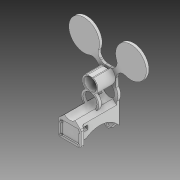
# Autodesk Inventor part: VisionMount
Saved by Autodesk Inventor 2020 (Build 240168000, 168)
## iProperties
Created: 2020-09-30
Part Number: VisionMount
Material: Generic
Document SubType Name: Modeling
Designer: DDeGo
Density: 1 g/cm^3
Appearance: Default
Author: DDeGo
Autodesk Inventor part; units mm, degrees
ref_plane "YZ Plane" through (0, 0, 0) normal (1, 0, 0) x (0, 1, 0)
ref_plane "XZ Plane" through (0, 0, 0) normal (0, 1, 0) x (-1, 0, 0)
ref_plane "XY Plane" through (0, 0, 0) normal (0, 0, 1) x (1, 0, 0)
sketch "Sketch1" plane through (0, 0, 0) normal (0, 0, 1) x (1, 0, 0)
  line L0 (-9.525, 7.14375) -> (-9.525, 19.84375)
  arc A0 (-9.525, 7.14375) -> (-10.31875, -5.939881) centre (0, 0) ccw
  line L1 (-10.31875, -5.939881) -> (-10.31875, -32.816122)
  line L2 (10.31875, -32.816122) -> (10.31875, -5.939881)
  arc A1 (10.31875, -5.939881) -> (9.525, 7.14375) centre (0, 0) ccw
  line L3 (9.525, 19.84375) -> (9.525, 7.14375)
  line L4 (5.55625, 23.8125) -> (9.525, 19.84375)
  line L5 (-9.525, 19.84375) -> (-5.55625, 23.8125)
  line L6 (-5.55625, 23.8125) -> (5.55625, 23.8125)
  line L7 (-10.31875, -32.816122) -> (10.31875, -32.816122)
  arc A2 (-9.525, 7.14375) -> (-10.31875, -5.939881) centre (0, 0) ccw
  arc A3 (10.31875, -5.939881) -> (9.525, 7.14375) centre (0, 0) ccw
  line L8 (0, -32.816122) -> (0, -23.019122) construction
  circle A4 centre (0, -23.019122) radius 2.75 construction
  circle A5 centre (0, 0) radius 8.05
  line L9 (-9.525, 7.14375) -> (10.31875, -5.939881) construction
  line L10 (-10.31875, -5.939881) -> (9.525, 7.14375) construction
  line L11 (9.525, 7.14375) -> (-9.525, 7.14375) construction
  line L12 (-10.31875, -5.939881) -> (10.31875, -5.939881) construction
  line L13 (-9.525, 19.84375) -> (9.525, 19.84375) construction
  line L14 (0, 0.863607) -> (0, 0) construction
  dimension "d0" = 20.6375
  dimension "d2" = 32.81612
  dimension "d3" = 23.8125
  dimension "d4" = 3.96875
  dimension "d5" = 19.05
  dimension "d6" = 9.797
  dimension "d7" = 5.5
  dimension "d8" = 16.1
  dimension "d69" = 11.90625
  dimension "d70" = 45
  dimension "d71" = 45
  dimension "d72" = 26.87624
  constraints: 30 end point, 8 point on circle, 6 centre point, 4 coincident, 4 horizontal, 4 vertical, 2 point on line, 1 concentric, 1 equal length, 1 midpoint, 1 parallel
  measures "d0" distance between parallel lines of L2 L1
  measures "d2" distance from line of L14.end L7
  measures "d3" distance from line of L6 L14.end
  measures "d4" distance from line of L6 L3.start
  measures "d5" distance between parallel lines of L3 L0
  measures "d6" distance of L8.start L8.end
  measures "d7" diameter of A4
  measures "d8" diameter of A5
  measures "d69" radius of A1
  measures "d70" angle of L13 L5
  measures "d71" angle of L13 L4
  measures "d72" distance between parallel lines of L7 L12
extrude "Extrusion1" add sketch "Sketch1" along normal blind 3
sketch "Sketch2" plane through (0, 0, 3) normal (0, 0, 1) x (1, 0, 0)
  line L0 (5.55625, 23.8125) -> (-5.55625, 23.8125)
  line L1 (0, 23.8125) -> (0, 15.8125) construction
  circle A0 centre (0, 15.8125) radius 7.05
  circle A1 centre (0, 0) radius 8.05
  arc A2 (-4.123106, 23.8125) -> (-3.182788, 7.394076) centre (0, 15.8125) ccw
  arc A3 (3.182788, 7.394076) -> (4.123106, 23.8125) centre (0, 15.8125) ccw
  point P0 (0, 0)
  dimension "d11" = 14.1
  dimension "d13" = 8
  dimension "d14" = 9
  constraints: 6 point on circle, 3 centre point, 2 coincident, 2 end point, 2 point on line, 1 concentric, 1 midpoint, 1 vertical
  measures "d11" diameter of A0
  measures "d13" distance of L1.start L1.end
  measures "d14" radius of A3
extrude "Extrusion2" add sketch "Sketch2" along normal blind 20 contours A3 A1 A2 L0
sketch "Sketch3" plane through (10.31875, -32.816122, 0) normal (1, 0, 0) x (0, 0, -1)
  line L0 (-3, 0) -> (-3, 26.876241)
  line L1 (-3, 5) -> (0, 2)
  line L2 (0, 0) -> (0, 26.876241)
  line L3 (0, 0) -> (-3, 0)
  line L4 (0, 2) -> (0, 0)
  line L5 (0, 0) -> (-3, 0)
  line L6 (-3, 5) -> (-3, 0)
  line L7 (-3, 7.047) -> (-3, 12.547)
  point P0 (0, 32.816122)
  dimension "d17" = 45
  dimension "d18" = 2
  constraints: 8 end point, 2 point on line, 1 collinear, 1 perpendicular, 1 vertical
  measures "d17" angle of L0 L1
  measures "d18" distance from line of L3 L1.end
extrude "Extrusion3" cut sketch "Sketch3" against normal through all
sketch "Sketch4" plane through (-5.55625, 23.8125, 0) normal (0, 1, 0) x (1, 0, 0)
  line L0 (13.60625, -3) -> (-2.49375, -3)
  line L1 (2.433144, -3) -> (8.679356, -3)
  line L2 (8.679356, -3) -> (8.679356, -5.5)
  line L3 (8.679356, -5.5) -> (2.433144, -5.5)
  line L4 (2.433144, -5.5) -> (2.433144, -3)
  line L5 (1.433144, -3) -> (1.433144, -23)
  line L6 (9.679356, -3) -> (9.679356, -23)
  point P0 (5.55625, 0)
  point P1 (8.739038, -3)
  point P2 (2.373462, -3)
  dimension "d21" = 1
  dimension "d22" = 1
  dimension "d23" = 2.5
  constraints: 8 end point, 2 parallel, 1 horizontal, 1 perpendicular, 1 point on line
  measures "d21" distance between parallel lines of L5 L4
  measures "d22" distance between parallel lines of L6 L2
  measures "d23" distance between parallel lines of L0 L3
extrude "Extrusion4" cut sketch "Sketch4" against normal blind 7.75
sketch "Sketch5" plane through (0, 0, 3) normal (0, 0, 1) x (1, 0, 0)
  arc A0 (-3.182788, 7.394076) -> (3.182788, 7.394076) centre (0, 0) ccw
  line L0 (-10.31875, -5.939881) -> (-10.31875, -30.816122)
  line L1 (10.31875, -27.816122) -> (10.31875, -5.939881)
  line L2 (-10.31875, -12.5) -> (10.31875, -12.5)
  line L3 (10.31875, -12.5) -> (10.31875, -9.5)
  line L4 (10.31875, -9.5) -> (-10.31875, -9.5) construction
  line L5 (-10.31875, -9.5) -> (-10.31875, -12.5)
  line L6 (-10.31875, -9.5) -> (-5.922314, -5.452403)
  line L7 (0, 0) -> (5.922314, -5.452403) construction
  line L8 (-5.922314, -5.452403) -> (0, 0) construction
  line L9 (5.922314, -5.452403) -> (10.31875, -9.5)
  point P0 (0, 0)
  point P1 (-10.31875, -9.5)
  dimension "d26" = 9.5
  dimension "d27" = 3
  constraints: 16 end point, 2 collinear, 2 parallel, 2 point on circle, 2 point on line, 1 horizontal, 1 perpendicular
  measures "d26" distance from line of point (0, 0) L4
  measures "d27" distance between parallel lines of L4 L2
extrude "Extrusion5" add sketch "Sketch5" along normal blind 40
sketch "Sketch7" plane through (0, 0, 43) normal (0, 0, 1) x (1, 0, 0)
  line L0 (-10.31875, -9.5) -> (-10.31875, -12.5)
  line L1 (-10.31875, -9.5) -> (-13, -11.968504)
  line L2 (-13, -11.968504) -> (-13, -29.968504)
  line L3 (-13, -29.968504) -> (13, -29.968504)
  line L4 (13, -29.968504) -> (13, -11.968504)
  line L5 (10.31875, -12.5) -> (10.31875, -9.5)
  line L6 (13, -11.968504) -> (10.31875, -9.5)
  arc A0 (-5.922314, -5.452403) -> (5.922314, -5.452403) centre (0, 0) ccw
  line L7 (10.31875, -9.5) -> (5.922314, -5.452403)
  line L8 (5.922314, -5.452403) -> (-5.922314, -5.452403) construction
  line L9 (-5.922314, -5.452403) -> (-10.318599, -9.499861)
  line L10 (-5.922314, -5.452403) -> (-10.31875, -9.5)
  arc A1 (-5.922314, -5.452403) -> (5.922314, -5.452403) centre (0, 0) ccw
  line L11 (-13, -11.968504) -> (13, -11.968504) construction
  point P0 (0, 0)
  dimension "d33" = 18
  dimension "d34" = 26
  constraints: 18 end point, 3 perpendicular, 2 collinear, 2 point on circle, 1 centre point, 1 concentric, 1 equal length, 1 horizontal, 1 parallel, 1 point on line
  measures "d33" distance between parallel lines of L3 L11
  measures "d34" distance of L1.end L4.end
extrude "Extrusion7" add sketch "Sketch7" along normal blind 3
sketch "Sketch9" plane through (10.31875, -5.939881, 3) normal (1, 0, 0) x (0, 0, -1)
  line L0 (0, -21.876241) -> (3, -24.876241)
  line L1 (-40, -6.028623) -> (-40, -24.028623)
  arc A0 (0, -21.876241) -> (-40, -24.028623) centre (-19.033714, -40.909955) ccw
  line L2 (0, -6.560119) -> (-40, -6.560119)
  line L3 (0, -21.876241) -> (0, -6.560119)
  point P0 (3, 5.939881)
  constraints: 2 point on circle, 1 centre point, 1 tangent
extrude "Extrusion8" add sketch "Sketch9" against normal blind 2
mirror "Mirror2" about plane through (0, 0, 0) normal (1, 0, 0) of "Extrusion8"
fillet "Fillet2" radius 2.5 2 edges at (10.3188, -19.7343, 43) (-10.3188, -19.7343, 43)
sketch "Sketch8" plane through (0, 0, 46) normal (0, 0, 1) x (1, 0, 0)
  line L0 (0, -29.968504) -> (0, -21.218504) construction
  line L1 (-10.25, -27.468504) -> (10.25, -27.468504) construction
  line L2 (10.25, -27.468504) -> (10.25, -14.968504) construction
  line L3 (10.25, -14.968504) -> (-10.25, -14.968504) construction
  line L4 (-10.25, -14.968504) -> (-10.25, -27.468504) construction
  line L5 (-10.25, -27.468504) -> (10.25, -14.968504) construction
  line L6 (10.25, -27.468504) -> (-10.25, -14.968504) construction
  circle A0 centre (-10.25, -14.968504) radius 1.2
  circle A1 centre (-10.25, -27.468504) radius 1.2
  circle A2 centre (10.25, -27.468504) radius 1.2
  circle A3 centre (10.25, -14.968504) radius 1.2
  line L7 (-13, -29.968504) -> (13, -29.968504)
  point P0 (0, 0)
  dimension "d37" = 2.4
  dimension "d38" = 12.5
  dimension "d39" = 20.5
  dimension "d40" = 2.5
  constraints: 14 end point, 4 centre point, 4 coincident, 3 equal radius, 3 midpoint, 2 parallel, 1 horizontal, 1 perpendicular, 1 vertical
  measures "d37" diameter of A1
  measures "d38" distance of L3.end L1.start
  measures "d39" distance of L1.start L2.start
  measures "d40" distance between parallel lines of L7 L1
extrude "Extrusion9" cut sketch "Sketch8" against normal blind 10
chamfer "Chamfer1" distance 12 angle 45 1 edges at (0, -12.5, 43)
sketch "Sketch10" plane through (0, 0, 36) normal (0, 0, 1) x (1, 0, 0)
  circle A0 centre (10.25, -14.968504) radius 1.2
  line L0 (12.35, -13.756068) -> (12.35, -16.18094)
  line L1 (12.35, -16.18094) -> (10.25, -17.393375)
  line L2 (10.25, -17.393375) -> (8.15, -16.18094)
  line L3 (8.15, -16.18094) -> (8.15, -13.756068)
  line L4 (8.15, -13.756068) -> (10.25, -12.543633)
  line L5 (10.25, -12.543633) -> (12.35, -13.756068)
  circle A1 centre (10.25, -27.468504) radius 1.2
  line L6 (12.35, -28.68094) -> (10.25, -29.893375)
  line L7 (10.25, -29.893375) -> (8.15, -28.68094)
  line L8 (8.15, -28.68094) -> (8.15, -26.256068)
  line L9 (8.15, -26.256068) -> (10.25, -25.043633)
  line L10 (10.25, -25.043633) -> (12.35, -26.256068)
  line L11 (12.35, -26.256068) -> (12.35, -28.68094)
  circle A2 centre (-10.25, -27.468504) radius 1.2
  line L12 (-12.35, -28.68094) -> (-12.35, -26.256068)
  line L13 (-12.35, -26.256068) -> (-10.25, -25.043633)
  line L14 (-10.25, -25.043633) -> (-8.15, -26.256068)
  line L15 (-8.15, -26.256068) -> (-8.15, -28.68094)
  line L16 (-8.15, -28.68094) -> (-10.25, -29.893375)
  line L17 (-10.25, -29.893375) -> (-12.35, -28.68094)
  arc A3 (-10.31875, -16.166533) -> (-10.31875, -13.770475) centre (-10.25, -14.968504) ccw
  line L18 (-12.35, -13.756068) -> (-10.25, -12.543633)
  line L19 (-10.25, -12.543633) -> (-8.15, -13.756068)
  line L20 (-8.15, -13.756068) -> (-8.15, -16.18094)
  line L21 (-8.15, -16.18094) -> (-10.25, -17.393375)
  line L22 (-10.25, -17.393375) -> (-12.35, -16.18094)
  line L23 (-12.35, -16.18094) -> (-12.35, -13.756068)
  point P0 (0, 0)
  dimension "d46" = 4.2
  constraints: 48 end point, 4 coincident, 4 vertical, 3 equal length, 52 other
  measures "d46" distance between parallel lines of L22 L19
extrude "Extrusion10" cut sketch "Sketch10" along normal up to surface (7 mm away) contours A0 | L0 L1 L2 L3 L4 L5 | A1 | L6 L7 L8 L9 L10 L11 | A2 | L12 L13 L14 L15 L16 L17 | L18 L19 L20 L21 L22 L23
sketch "Sketch11" plane through (0, 0, 43) normal (0, 0, -1) x (-1, 0, 0)
  line L0 (-14.400225, -28.68094) -> (18.488326, -28.68094)
  line L1 (18.488326, -28.68094) -> (18.488326, -34.634031)
  line L2 (18.488326, -34.634031) -> (-14.400225, -34.634031)
  line L3 (-14.400225, -34.634031) -> (-14.400225, -28.68094)
  point P0 (0, 0)
  point P1 (12.35, -28.68094)
  constraints: 8 end point, 2 parallel, 1 horizontal, 1 perpendicular, 1 point on line
extrude "Extrusion11" cut sketch "Sketch11" along normal blind 10
sketch "Sketch12" plane through (0, 0, 46) normal (0, 0, 1) x (1, 0, 0)
  circle A0 centre (-10.25, -27.468504) radius 1.2 construction
  line L0 (-10.25, -27.468504) -> (10.25, -27.468504)
  line L1 (10.25, -27.468504) -> (10.25, -11.968504)
  line L2 (10.25, -11.968504) -> (-10.25, -11.968504)
  line L3 (-10.25, -11.968504) -> (-10.25, -27.468504)
  circle A1 centre (10.25, -27.468504) radius 1.2 construction
  circle A2 centre (-10.25, -14.968504) radius 1.2
  point P0 (0, 0)
  point P1 (-10.25, -13.768504)
  point P2 (-10.25, -16.168504)
  dimension "d51" = 3
  constraints: 8 end point, 2 parallel, 1 coincident, 1 horizontal, 1 perpendicular
  measures "d51" distance from line of A2.centre L2
extrude "Extrusion12" cut sketch "Sketch12" against normal blind 1.5 contours L3 A2 L2 L1 L0
fillet "Fillet3" radius 2.5 4 edges at (13, -29.9685, 44.5) (-13, -29.9685, 44.5) (13, -11.9685, 44.5) (-13, -11.9685, 44.5)
sketch "Sketch13" plane through (0, 0, 0) normal (0, 0, -1) x (-1, 0, 0)
  line L0 (0, 0) -> (0, 79.709992) construction
  line L1 (-5.55625, 23.8125) -> (5.55625, 23.8125)
  line L2 (5.55625, 23.8125) -> (9.525, 19.84375)
  line L3 (5.55625, 23.8125) -> (9.525, 19.84375)
  line L4 (9.525, 19.84375) -> (16.40266, 26.72141)
  line L5 (28.616883, 38.935633) -> (24.648133, 42.904383) construction
  line L6 (24.648133, 42.904383) -> (12.43391, 30.69016) construction
  arc A0 (16.40266, 26.72141) -> (12.43391, 30.69016) centre (26.632508, 40.920008) ccw
  line L7 (12.43391, 30.69016) -> (5.55625, 23.8125)
  line L8 (16.40266, 26.72141) -> (28.616883, 38.935633) construction
  arc A1 (12.43391, 30.69016) -> (16.40266, 26.72141) centre (26.632508, 40.920008) ccw construction
  line L9 (-5.55625, 23.8125) -> (-9.525, 19.84375)
  line L10 (-5.55625, 23.8125) -> (-9.525, 19.84375)
  line L11 (-9.525, 19.84375) -> (-16.40266, 26.72141)
  line L12 (-28.616883, 38.935633) -> (-24.648133, 42.904383) construction
  line L13 (-24.648133, 42.904383) -> (-12.43391, 30.69016) construction
  arc A2 (-12.43391, 30.69016) -> (-16.40266, 26.72141) centre (-26.632508, 40.920008) ccw
  line L14 (-12.43391, 30.69016) -> (-5.55625, 23.8125)
  line L15 (-16.40266, 26.72141) -> (-28.616883, 38.935633) construction
  arc A3 (-16.40266, 26.72141) -> (-12.43391, 30.69016) centre (-26.632508, 40.920008) ccw construction
  dimension "d58" = 27
  dimension "d59" = 35
  constraints: 28 end point, 8 point on circle, 6 symmetric about line, 5 parallel, 4 centre point, 2 perpendicular, 1 collinear, 1 midpoint, 1 vertical, 2 other
  measures "d58" distance between parallel lines of L2 L5
  measures "d59" diameter of A0
extrude "Extrusion13" add sketch "Sketch13" against normal up to surface (3 mm away)
fillet "Fillet4" radius 7 8 edges at (16.4027, 26.7214, 1.5) (9.525, 19.8438, 1.5) (5.5562, 23.8125, 1.5) (12.4339, 30.6902, 1.5) (-5.5563, 23.8125, 1.5) (-12.4339, 30.6902, 1.5) (-9.525, 19.8438, 1.5) (-16.4027, 26.7214, 1.5)
sketch "Sketch14" plane through (0, 0, 23) normal (0, 0, 1) x (1, 0, 0)
  circle A0 centre (0, 0) radius 8.05
  circle A1 centre (0, 0) radius 10.05
  circle A2 centre (0, 15.8125) radius 7.05 projected
  point P0 (-3.182788, 7.394076)
  point P1 (3.195683, 9.528384)
  point P2 (-3.195683, 9.528384)
  dimension "d66" = 2
  constraints: 2 coincident, 1 centre point, 3 other
extrude "Extrusion14" add sketch "Sketch14" against normal blind 3 contours A1 A2 picked at (9.201681, 1.469149)
chamfer "Chamfer2" distance 0.5 angle 45 4 edges at (6.0097, 12.1265, 23) (-3.686, 21.8222, 23) (0, 8.7625, 23) (-8.05, 0, 0)
sketch "Sketch15" plane through (0, 0, 3) normal (0, 0, 1) x (1, 0, 0)
  line L0 (-8.31875, -27.816122) -> (8.31875, -27.816122)
  line L1 (0, -27.816122) -> (0, -33.816122) construction
  circle A0 centre (0, -33.816122) radius 1.75
  arc A1 (-3.304487, -36.488735) -> (3.304487, -36.488735) centre (0, -33.816122) ccw
  line L2 (-10.31875, -27.816122) -> (-8.31875, -27.816122)
  line L3 (-10.31875, -27.816122) -> (-3.304487, -36.488735)
  line L4 (8.31875, -27.816122) -> (10.31875, -27.816122)
  line L5 (3.304487, -36.488735) -> (10.31875, -27.816122)
  line L6 (10.31875, -27.816122) -> (-10.31875, -27.816122)
  point P0 (0, 0)
  dimension "d73" = 6
  dimension "d74" = 3.5
  dimension "d75" = 2.5
  constraints: 8 end point, 2 centre point, 2 coincident, 2 point on circle, 2 tangent, 1 collinear, 1 midpoint, 1 vertical
  measures "d73" distance of L1.start L1.end
  measures "d74" diameter of A0
  measures "d75" radial gap between concentric circles of A0 A1
extrude "Extrusion15" add sketch "Sketch15" against normal up to surface (3 mm away)
chamfer "Chamfer3" distance 1 distance2 3 3 edges at (0, -38.0661, 3) (6.8116, -32.1524, 3) (-6.8116, -32.1524, 3) measured on face at (-6.4229, -31.838, 3) measured on face at (0, -37.5661, 3) measured on face at (6.4229, -31.838, 3)
body "Solid1"
